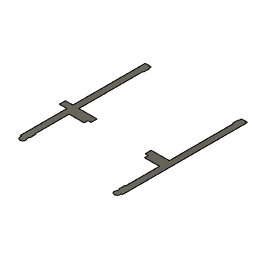
1F廊下用平面[少し幅大きく作ったから修正入れていこう] (Autodesk Fusion 360 design; units mm, degrees)
Autodesk Fusion 360 part; units mm, degrees
sketch "スケッチ1" plane through (0, 0, 0) normal (0, 0, 1) x (1, 0, 0)
  line L0 (0, -4000) -> (0, -35000)
  line L1 (-4000, -6500.036) -> (-14000, -6500.036)
  line L2 (-34000, 2000) -> (-34000, -2000)
  line L3 (-63500, -29000.036) -> (-64000, -29000.036)
  line L4 (-63500, 42500) -> (-63500, 46500)
  line L5 (-64000, 46500) -> (-64000, 48000)
  line L6 (-64000, -6500.036) -> (-64000, -29000.036)
  line L7 (-14000, -6500.036) -> (-14000, -4000)
  line L8 (-68000, 41000) -> (-68000, 43977.4822)
  arc A0 (-67000, -35000) -> (-64000, -34500.036) centre (-65310.0198, -35889.9814) ccw
  line L9 (-1000, -35000) -> (0, -35000)
  arc A1 (-4000, -34500.036) -> (-1000, -35000) centre (-2689.9802, -35889.9814) ccw
  line L10 (-67000, -35000) -> (-68000, -35000)
  line L11 (-4000, 46500) -> (-4000, 48000)
  line L12 (-68000, 0) -> (-68000, 41000)
  line L13 (0, 41000) -> (0, 43977.4822)
  line L14 (-63500, 46500) -> (-64000, 46500)
  line L15 (-4500, 46500) -> (-4000, 46500)
  line L16 (-64000, 42500) -> (-63500, 42500)
  line L17 (-4000, -33000.036) -> (-4500, -33000.036)
  line L18 (-68000, 43977.4822) -> (-68000, 48000)
  line L19 (-68000, 48000) -> (-64000, 48000)
  line L20 (-78000, 0) -> (-79000, 0)
  line L21 (10000, 0) -> (11000, 0)
  line L22 (-64000, -6500.036) -> (-54000, -6500.036)
  line L23 (-63500, -33000.036) -> (-63500, -29000.036)
  line L24 (-64000, -34500.036) -> (-64000, -33000.036)
  line L25 (-64000, -33000.036) -> (-63500, -33000.036)
  line L26 (-68000, -4000) -> (-68000, -35000)
  line L27 (0, 0) -> (0, 41000)
  line L28 (-64000, 0) -> (-64000, 42500)
  line L29 (-54000, -6500.036) -> (-54000, -4000)
  line L30 (-4500, 42500) -> (-4500, 46500)
  line L31 (-4000, 42500) -> (-4500, 42500)
  line L32 (-4500, -29000.036) -> (-4000, -29000.036)
  line L33 (-4000, 0) -> (-4000, 42500)
  line L34 (-4500, -33000.036) -> (-4500, -29000.036)
  line L35 (-4000, -34500.036) -> (-4000, -33000.036)
  line L36 (0, 48000) -> (-4000, 48000)
  line L37 (-4000, -6500.036) -> (-4000, -29000.036)
  line L38 (0, 43977.4822) -> (0, 48000)
  line L39 (-64000, 0) -> (-52000, 0)
  line L40 (-52000, 0) -> (-52000, -4000)
  line L41 (-54000, -4000) -> (-52000, -4000)
  line L42 (-4000, 0) -> (-16000, 0)
  line L43 (-16000, 0) -> (-16000, -4000)
  line L44 (-16000, -4000) -> (-14000, -4000)
  line L45 (0, -4000) -> (0, 0)
  line L46 (-73000, 0) -> (-73000, -4000)
  line L47 (-73000, 0) -> (-68000, 0)
  line L48 (-68000, -4000) -> (-73000, -4000)
  point P0 (-4000, -35000)
  point P1 (-64000, -35000)
  point P2 (-64000, 42500)
  point P3 (-64000, -34500.036)
  point P4 (-68000, 0)
  point P5 (-64000, -6500.036)
  point P6 (-64000, 0)
  point P7 (-4000, 0)
  point P8 (-4000, 41000)
  point P9 (-4000, 42500)
  point P10 (-4000, -6500.036)
  point P11 (-4000, -34500.036)
  point P12 (-64000, 0)
  point P13 (-64000, 41000)
  constraint parallel L8 L18
  constraint perpendicular L5 L14
  constraint perpendicular L11 L15
  constraint perpendicular L15 L38
  constraint perpendicular L11 L36
  constraint perpendicular L5 L19
  constraint coincident P12 P6
  constraint perpendicular L28 L39
  constraint perpendicular L40 L41
  constraint coincident P7 L33.start
  constraint perpendicular L33 L42
  constraint perpendicular L7 L44
  constraint perpendicular L42 L45
  constraint perpendicular L46 L47
  constraint perpendicular L46 L48
extrude "押し出し1" add sketch "スケッチ1" along normal blind 10 makes body 1 at (-60666.6667, -3500.012, 0) makes body 2 at (-7333.3333, -3500.012, 0)
